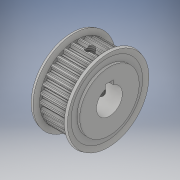
# Autodesk Inventor part: HTPA30S3M100-A-N10_b
Saved by Autodesk Inventor 2019 (Build 230136000, 136)
## iProperties
Created: 2022-11-15
Part Number: HTPA30S3M100-A-N10_b
Material: Generic
Catalog Web Link: www.cadenas.de
Description: HTPA__S3M060, HTPA__S3M100, HTPA__S3M150, HTPB__S3M060, HTPB__S3M100, HTPB__S3M150, HTPK__S3M060, HTPK__S3M100, HTPK__S3M150, HTPN__S3M060, HTPN__S3M100, HTPN__S3M150, HTPT__S3M060, HTPT__S3M100, HTPT__S3M150, HTPM__S3M060, HTPM__S3M100, HTPM__S3M150, HTPP__S3M060, HTPP__S3M100, HTPP__S3M150, HTPS__S3M060, HTPS__S3M100, KHTPA__S3M060, KHTPA__S3M100, KHTPA__S3M150, KHTPK__S3M060, KHTPK__S3M100, KHTPK__S3M150_body-High Torque Timing Pulleys S3M Type
Vendor: MISUMI
Document SubType Name: Modeling
Designer: psAdmin
Manufacturer: MISUMI
Mass: 7.23105 g
Surface Area: 42.2616 cm^2
Volume: 7.23105 cm^3
Density: 1 g/cm^3
Appearance: PSOLRGB-175-175-175
Category: PARTsolutions
Company: MISUMI
Title: HTPA30S3M100-A-N10
Author: Cadenas PARTsolutions
Comments: High Torque Timing Pulleys S3M Type
PSOL_IDENT_0: {$CADENAS_DATA/23d-libs/misumi/metric/51_timing_pulleys/htpk_s3m/htpa_s3m.prj},837 {VTYP=3D},{NB=HTP
PSOL_IDENT_1: A30S3M100-A-N10_b},{LINA=HTPA30S3M100-A-N10},{NN=HTPA__S3M060, HTPA__S3M100, HTPA__S3M150, HTPB__S3M
PSOL_IDENT_2: 060, HTPB__S3M100, HTPB__S3M150, HTPK__S3M060, HTPK__S3M100, HTPK__S3M150, HTPN__S3M060, HTPN__S3M10
PSOL_IDENT_3: 0, HTPN__S3M150, HTPT__S3M060, HTPT__S3M100, HTPT__S3M150, HTPM__S3M060, HTPM__S3M100, HTPM__S3M150,
PSOL_IDENT_4: HTPP__S3M060, HTPP__S3M100, HTPP__S3M150, HTPS__S3M060, HTPS__S3M100, KHTPA__S3M060, KHTPA__S3M100,
PSOL_IDENT_5: KHTPA__S3M150, KHTPK__S3M060, KHTPK__S3M100, KHTPK__S3M150_body},{DATE=28.10.2022 00:10:57},{GEOMDA
PSOL_IDENT_6: TE=11.11.2021 09:52:43},{VERSION=},{LINEID=160},{WBVAR=MATP,ST,TNW,PS,SBS,DD,Z,J,Q,R,S,T,ALT1,ALT2,M
PSOL_IDENT_7: ,QSC,QFC,QTC,ALT3,K,KSC,KFC,KTC,ALT4,ZM,ZSC,ZFC,ZTC,ALT5,ALT6,ALT7,FC,ALT8,SRG,ALT9,BTC,TL,ALT10,TPC
PSOL_IDENT_8: ,ALT11,BC,ALT12,SLH,ALT13,BN},{WBNUMERIC=DD,Z,J,Q,R,S,T,QSC,QFC,QTC,K,KSC,KFC,KTC,ZSC,ZFC,ZTC,FC,SRG
PSOL_IDENT_9: ,BTC,TL,BC,SLH,BN}  {NB=HTPA30S3M100-A-N10_b},{LINA=HTPA30S3M100-A-N10},{KT=DUMMY},{PN=HTPA30S3M100-
PSOL_IDENT_10: A-N10},{TYPE=HTPA},{MATP=A2017},{MATPALG='A2017','Aluminum Alloy 2000 series','S45C','1045 Carbon St
PSOL_IDENT_11: eel Equivalent','SUS304','304 Stainless Steel','A6000','6000 Series Aluminum Alloy'},{ST=CA},{STALG=
PSOL_IDENT_12: 'CA','Clear Anodize','BA','Black Anodize','HAT','Hard Clear Anodize','ENP','Electroless Nickel Plat
PSOL_IDENT_13: ing' },{NT=30},{TNW=S3M100},{TNWALG= 'S3M060','S3M100','S3M150'    },{BW=10},{PS=A},{PSALG='A','B'},
PSOL_IDENT_14: {SBS=N},{SBSALG= 'H','Round Hole','P','Round Hole + Tap','N','New JIS Keywayed Bore + Tap (Standard)'
PSOL_IDENT_15: ,'NK','New JIS Keywayed Bore + Tap (width 4.0mm, height 1.8mm)','C','Old JIS Keywayed Bore + Tap','V'
PSOL_IDENT_16: ,'Stepped Hole', 'Y','Both Ends Stepped Hole','WB', 'Double Stepped Hole' },{SHSA= 'H','Round Hole','
PSOL_IDENT_17: P','Round Hole + Tap','N','New JIS Keywayed Bore + Tap (Standard)','NK','New JIS Keywayed Bore + Tap
PSOL_IDENT_18: (width 4.0mm, height 1.8mm)','C','Old JIS Keywayed Bore + Tap','V','Stepped Hole', 'Y','Both Ends S
PSOL_IDENT_19: tepped Hole','WB', 'Double Stepped Hole' },{SHSB= 'H','Round Hole','P','Round Hole + Tap','N','New J
PSOL_IDENT_20: IS Keywayed Bore + Tap (Standard)','NK','New JIS Keywayed Bore + Tap (width 4.0mm, height 1.8mm)','C'
PSOL_IDENT_21: ,'Old JIS Keywayed Bore + Tap','V','Stepped Hole', 'F','Stepped Hole (Counterbore holes on the boss
PSOL_IDENT_22: side)'},{SHSK= '','' },{SBSPN=-N10},{DD=10.00},{DDALG=[8:8/1],[10:14/1]},{DDHA=[6:6/1],6.35,[7:12/1]
PSOL_IDENT_23: ,12.7,[13:19/1]},{DDHBK=0},{DDPA=[6:6/1],6.35,[7:12/1],12.7,[13:19/1]},{DDPBK=0},{DDNA=[8:8/1],[10:1
PSOL_IDENT_24: 4/1]},{DDNBK=0},{DDNK=10},{DDCA=[10:10/1],[12:12/1]},{DDCBK=0},{DDVA=[6:6/1],6.35,[7:12/1],12.7,[13:
PSOL_IDENT_25: 17/1]},{DDVF=[6:6/1],6.35,[7:12/1],12.7,[13:14/1]},{DDY=[6:17/1]},{DDWB=[6:15/1]},{Z=0},{ZALG=[0]},{
PSOL_IDENT_26: ZQRMIN=12},{ZAMAX=19},{ZBMAX=16},{DDZ=10},{J=0.0},{JALG=[0]},{JMAX=13},{JMIN=2},{JPN=},{QRMAX=19},{Q
PSOL_IDENT_27: RMIN=12},{WBRMAX=-2.00},{WBQMIN=14},{Q=0},{QALG=[0]},{QPN=},{R=0},{RALG=[0]},{S=0.0},{SALG=[0]},{SPN=
PSOL_IDENT_28: },{SMAX=9},{T=0.0},{TALG=[0]},{TPN=},{TMAX=12},{A=11},{W=15},{L=0},{PD=28.65},{OD=27.89},{D=0},{DALG=
PSOL_IDENT_29: 20},{DE=23},{F=32},{E=23},{BBK=3.000},{TTK=1.4},{TT=1},{ANG=120},{WL=15},{ALT1=},{ALT1ALG= '','w/o K
PSOL_IDENT_30: C90 (Set Screw Angle)','KC90','with KC90 (Set Screw Angle)' },{ALT1PN=},{ALT2=},{ALT2ALG= '','Not ap
PSOL_IDENT_31: plicable' },{M=N/A},{MALG= 'N/A' },{MFTALG= 'N/A' },{MSALG= 'N/A' },{M3D=0.000},{KDML=0},{ML=0},{MUL=
PSOL_IDENT_32: 0},{PITCH=0},{QSC=0.0},{QSCALG=0},{QFC=0.0},{QFCALG=0},{QTC=0.0},{QTCALG=0},{QPCDMIN=0},{QPCDMINALG=
PSOL_IDENT_33: 0},{QPCDMAX=19},{ALT2PN=},{ALT3=},{ALT3ALG= '','Not applicable' },{K=0.0},{KALG=0},{KMIN=4},{KFTMAX=
PSOL_IDENT_34: 0.0},{KSMAX=0.0},{KSC=0.0},{KSCALG=0},{KFC=0.0},{KFCALG=0},{KTC=0.0},{KTCALG=0},{KPCDMIN=14},{KPCDMI
PSOL_IDENT_35: NALG=14},{KPCDMAX=19},{KSCMIN=14.0},{KSCMINALG=14},{ALT3PN=},{ALT4=},{ALT4ALG= '','Not applicable' }
PSOL_IDENT_36: ,{ALT4MIN=20.5},{ALT4MAX=12.5},{ZM=N/A},{ZMALG= 'N/A' },{ZMSALG= 'N/A' },{ZMFTALG= 'N/A' },{ZMDD1=0.
PSOL_IDENT_37: 0},{ZMDD2=0.0},{ZMHH=0.0},{ZSC=0.0},{ZSCALG=[0]},{ZFC=0.0},{ZFCALG=[0]},{ZTC=0.0},{ZTCALG=[0]},{ZPCD
PSOL_IDENT_38: MIN=0},{ZPCDMINALG=0},{ZPCDMAX=19},{ALT4PN=},{ALT5=},{ALT5ALG= '','Flange Attached','NFC','with NFC
PSOL_IDENT_39: (Flange not Attached)' },{ALT5PN=},{ALT6=},{ALT6ALG= '','w/o Flange Attached on One Side Only','RFC'
PSOL_IDENT_40: ,'with RFC (Flange Attached on The Boss Side Only)','LFC','with LFC (Flange Attached on The Opposite
PSOL_IDENT_41: Side Only)' },{ALT6PN=},{ALT7=},{ALT7ALG= '','w/o FC (Flange Cut)','FC','with FC (Flange Cut)' },{F
PSOL_IDENT_42: C=0.0},{FCALG=0},{FCMIN=29.0},{FCMAX=30.0},{ALT7PN=},{ALT8=},{ALT8ALG= '','Not applicable' },{ALT8AL
PSOL_IDENT_43: GALG=19},{ALT8DD2=0},{ALT8MM=0},{ALT8NN=0},{QC=0},{KC=0},{ZC=0},{SRG=0.0},{SRGALG=[0]},{SRGMAX1=0},{
PSOL_IDENT_44: SRGMAX=0},{DD2=0.0},{MM=0.00},{NN=0.00},{ALT8PN=},{ALT9ALG= '','Not applicable' },{ALT9=},{BTC9=11},
PSOL_IDENT_45: {TL9=1},{BTC=0},{BTCALG=[0]},{TL=0.0},{TLALG=0},{TLMIN=1.0},{TLMAX=-15.5},{BTCL=0},{BTCD=0},{BTCDALG=
PSOL_IDENT_46: 20.000},{ALT9PN=},{WLBCTL=15},{ALT10=},{ALT10ALG= '','w/o TPC (Tapped Hole Dimension)','TPC','with T
PSOL_IDENT_47: PC (Tapped Hole Dimension)' },{TPC=N/A},{TPCALG= 'N/A' },{TPCM=4},{ALT10PN=},{ALT11=},{ALT11ALG= '','
PSOL_IDENT_48: Not applicable' },{BC=0.0},{BCALG=0},{BCMIN=7},{BCMAX=-15.5},{BCPLANE=7.5},{M1WBC=7.5},{ALT11PN=},{A
PSOL_IDENT_49: LT12=},{ALT12ALG= '','w/o SLH (Set Screw Length)','SLH','with SLH (Set Screw Length)' },{SLH=0},{SLH
PSOL_IDENT_50: ALG=[0]},{ALT12PN=},{AC=M4x3},{M1=4},{M1L=3},{TAP=0.000},{KYY=5},{KTT=8.945},{PLANE=15},{CD=0},{ALT1
PSOL_IDENT_51: 3=},{ALT13ALG= '', 'Not applicable' },{BN=0.0},{BNALG=0},{BNMIN=-14.5},{BNMAX=-5.0},{ALT13PN=}
NB: HTPA30S3M100-A-N10_b
NN: 0
NT: 30
NBSYN: $PN._b
LINA: HTPA30S3M100-A-N10
CATALOG: Misumi
PN: HTPA30S3M100-A-N10
MATP: Aluminum Alloy 2000 series
ST: Clear Anodize
TNW: S3M100
BW: 10
PS: A
SBS: New JIS Keywayed Bore + Tap (Standard)
DD: 10
Z: 0
J: 0
Q: 0
R: 0
S: 0
T: 0
A: 11
W: 15
L: 0
PD: 28.65
OD: 27.89
D: 0
F: 32
E: 23
TT: 1
ALT1: w/o KC90 (Set Screw Angle)
ALT2: Not applicable
M: N/A
QSC: 0
QFC: 0
QTC: 0
ALT3: Not applicable
K: 0
KSC: 0
KFC: 0
KTC: 0
ALT4: Not applicable
ZM: N/A
ZMDD1: 0
ZMDD2: 0
ZMHH: 0
ZSC: 0
ZFC: 0
ZTC: 0
ALT5: Flange Attached
ALT6: w/o Flange Attached on One Side Only
ALT7: w/o FC (Flange Cut)
FC: 0
ALT8: Not applicable
SRG: 0
DD2: 0
MM: 0
ALT9: Not applicable
BTC: 0
TL: 0
BTCL: 0
BTCD: 0
ALT10: w/o TPC (Tapped Hole Dimension)
TPC: N/A
ALT11: Not applicable
BC: 0
ALT12: w/o SLH (Set Screw Length)
SLH: 0
AC: M4x3
ALT13: Not applicable
BN: 0
SUPPLIER: MISUMI
ARTICLENO: HTPA30S3M100-A-N10_b
BOMINFO: HTPA30S3M100-A-N10
CREATOR: CADENAS GmbH
Autodesk Inventor part; units mm, degrees
sketch "_____1" plane through (0, 0, 0) normal (0, 0, 1) x (1, 0, 0)
  line L0 (15, 0) -> (0, 0)
  line L1 (0, 0) -> (0, 11.5)
  line L2 (0, 11.5) -> (1, 11.5)
  line L3 (1, 11.5) -> (1, 13.813348)
  line L4 (1, 13.813348) -> (0.483439, 15.741181)
  line L5 (0.483439, 15.741181) -> (1.449364, 16)
  line L6 (1.449364, 16) -> (2, 13.945)
  line L7 (2, 13.945) -> (13, 13.945)
  line L8 (13, 13.945) -> (13.550636, 16)
  line L9 (13.550636, 16) -> (14.516561, 15.741181)
  line L10 (14.516561, 15.741181) -> (14, 13.813348)
  line L11 (14, 13.813348) -> (14, 11.5)
  line L12 (14, 11.5) -> (15, 11.5)
  line L13 (15, 11.5) -> (15, 0)
  line L14 (15, 0) -> (0, 0)
  constraints: 30 end point
revolve "Revolution1" add sketch "_____1" angle 360 about axis through (15, 0, 0) along (1, 0, 0)
sketch "Sketch2" plane through (15, 0, 0) normal (1, 0, 0) x (0, 0, -1)
  point P0 (0, 0)
hole "Hole1" at (15, 0, 0) direction (-1, 0, 0) diameter 10 depth 15
sketch "_____6" plane through (2, 0, 0) normal (1, 0, 0) x (0, 0, -1)
  circle A0 centre (0, 0) radius 18.945
  arc A1 (-13.942597, 0.258894) -> (-13.942597, -0.258894) centre (0, 0) ccw
  arc A2 (-13.942597, -0.258894) -> (-13.718388, -0.52809) centre (-13.662645, -0.253695) ccw
  arc A3 (-12.845232, -0.94797) -> (-13.718388, -0.52809) centre (-14.111574, -2.463557) ccw
  arc A4 (-12.791913, -1.050797) -> (-12.845232, -0.94797) centre (-12.94141, -1.063078) ccw
  arc A5 (-12.791913, -1.050797) -> (-12.730852, -1.631754) centre (0, 0) ccw
  arc A6 (-12.761627, -1.74342) -> (-12.730852, -1.631754) centre (-12.879635, -1.650824) ccw
  arc A7 (-13.528404, -2.335663) -> (-12.761627, -1.74342) centre (-14.315404, -0.524239) ccw
  arc A8 (-13.528404, -2.335663) -> (-13.691744, -2.645593) centre (-13.416829, -2.592472) ccw
  arc A9 (-13.691744, -2.645593) -> (-13.58409, -3.152065) centre (0, 0) ccw
  arc A10 (-13.58409, -3.152065) -> (-13.308812, -3.368764) centre (-13.311337, -3.088775) ccw
  arc A11 (-12.367439, -3.597928) -> (-13.308812, -3.368764) centre (-13.291, -5.343683) ccw
  arc A12 (-12.293906, -3.687423) -> (-12.367439, -3.597928) centre (-12.437583, -3.730517) ccw
  arc A13 (-12.293906, -3.687423) -> (-12.113392, -4.242989) centre (0, 0) ccw
  arc A14 (-12.120277, -4.358613) -> (-12.113392, -4.242989) centre (-12.254959, -4.292576) ccw
  arc A15 (-12.747165, -5.097336) -> (-12.120277, -4.358613) centre (-13.893583, -3.489123) ccw
  arc A16 (-12.747165, -5.097336) -> (-12.842497, -5.434454) centre (-12.584634, -5.325336) ccw
  arc A17 (-12.842497, -5.434454) -> (-12.631894, -5.907476) centre (0, 0) ccw
  arc A18 (-12.631894, -5.907476) -> (-12.317577, -6.062206) centre (-12.37826, -5.78886) ccw
  arc A19 (-11.349129, -6.09064) -> (-12.317577, -6.062206) centre (-11.889545, -7.990265) ccw
  arc A20 (-11.258597, -6.162891) -> (-11.349129, -6.09064) centre (-11.390174, -6.234915) ccw
  arc A21 (-11.258597, -6.162891) -> (-10.966518, -6.668785) centre (0, 0) ccw
  arc A22 (-10.949214, -6.783314) -> (-10.966518, -6.668785) centre (-11.094682, -6.746722) ccw
  arc A23 (-11.408813, -7.636232) -> (-10.949214, -6.783314) centre (-12.864545, -6.301516) ccw
  arc A24 (-11.408813, -7.636232) -> (-11.431971, -7.985803) centre (-11.20243, -7.825457) ccw
  arc A25 (-11.431971, -7.985803) -> (-11.127624, -8.404702) centre (0, 0) ccw
  arc A26 (-11.127624, -8.404702) -> (-10.788005, -8.4907) centre (-10.904194, -8.235945) ccw
  arc A27 (-9.834808, -8.317162) -> (-10.788005, -8.4907) centre (-9.968461, -10.287634) ccw
  arc A28 (-9.731232, -8.369011) -> (-9.834808, -8.317162) centre (-9.844959, -8.466818) ccw
  arc A29 (-9.731232, -8.369011) -> (-9.340355, -8.803124) centre (0, 0) ccw
  arc A30 (-9.299617, -8.911552) -> (-9.340355, -8.803124) centre (-9.449514, -8.906004) ccw
  arc A31 (-9.571841, -9.841387) -> (-9.299617, -8.911552) centre (-11.273265, -8.838502) ccw
  arc A32 (-9.571841, -9.841387) -> (-9.521814, -10.188135) centre (-9.330626, -9.983569) ccw
  arc A33 (-9.521814, -10.188135) -> (-9.137023, -10.534602) centre (0, 0) ccw
  arc A34 (-9.137023, -10.534602) -> (-8.786945, -10.54811) centre (-8.953562, -10.323079) ccw
  arc A35 (-7.890659, -10.180183) -> (-8.786945, -10.54811) centre (-7.611706, -12.135384) ccw
  arc A36 (-7.778566, -10.209365) -> (-7.890659, -10.180183) centre (-7.869473, -10.32868) ccw
  arc A37 (-7.778566, -10.209365) -> (-7.305974, -10.552723) centre (0, 0) ccw
  arc A38 (-7.243582, -10.650312) -> (-7.305974, -10.552723) centre (-7.391357, -10.676051) ccw
  arc A39 (-7.316534, -11.616427) -> (-7.243582, -10.650312) centre (-9.18929, -10.989203) ccw
  arc A40 (-7.316534, -11.616427) -> (-7.195507, -11.945196) centre (-7.051029, -11.70535) ccw
  arc A41 (-7.195507, -11.945196) -> (-6.74709, -12.20409) centre (0, 0) ccw
  arc A42 (-6.74709, -12.20409) -> (-6.401854, -12.144517) centre (-6.611616, -11.959045) ccw
  arc A43 (-5.60165, -11.598282) -> (-6.401854, -12.144517) centre (-4.922284, -13.45276) ccw
  arc A44 (-5.48594, -11.603521) -> (-5.60165, -11.598282) centre (-5.550053, -11.739129) ccw
  arc A45 (-5.48594, -11.603521) -> (-4.952286, -11.841118) centre (0, 0) ccw
  arc A46 (-4.870968, -11.923603) -> (-4.952286, -11.841118) centre (-5.010163, -11.979503) ccw
  arc A47 (-4.741459, -12.883773) -> (-4.870968, -11.923603) centre (-6.703698, -12.659623) ccw
  arc A48 (-4.741459, -12.883773) -> (-4.554722, -13.180195) centre (-4.463268, -12.915551) ccw
  arc A49 (-4.554722, -13.180195) -> (-4.062277, -13.3402) centre (0, 0) ccw
  arc A50 (-4.062277, -13.3402) -> (-3.736971, -13.210151) centre (-3.980711, -13.072344) ccw
  arc A51 (-3.067822, -12.50948) -> (-3.736971, -13.210151) centre (-2.017734, -14.182185) ccw
  arc A52 (-2.953551, -12.490547) -> (-3.067822, -12.50948) centre (-2.988069, -12.636521) ccw
  arc A53 (-2.953551, -12.490547) -> (-2.38216, -12.612) centre (0, 0) ccw
  arc A54 (-2.285469, -12.675775) -> (-2.38216, -12.612) centre (-2.41, -12.759394) ccw
  arc A55 (-1.959159, -13.588036) -> (-2.285469, -12.675775) centre (-3.925122, -13.776757) ccw
  arc A56 (-1.959159, -13.588036) -> (-1.714874, -13.839156) centre (-1.680441, -13.561281) ccw
  arc A57 (-1.714874, -13.839156) -> (-1.199923, -13.893279) centre (0, 0) ccw
  arc A58 (-1.199923, -13.893279) -> (-0.908764, -13.698437) centre (-1.17583, -13.614318) ccw
  arc A59 (-0.399916, -12.873954) -> (-0.908764, -13.698437) centre (0.975, -14.291781) ccw
  arc A60 (-0.292078, -12.831676) -> (-0.399916, -12.873954) centre (-0.295492, -12.981637) ccw
  arc A61 (-0.292078, -12.831676) -> (0.292078, -12.831676) centre (0, 0) ccw
  arc A62 (0.399916, -12.873954) -> (0.292078, -12.831676) centre (0.295492, -12.981637) ccw
  arc A63 (0.908764, -13.698437) -> (0.399916, -12.873954) centre (-0.975, -14.291781) ccw
  arc A64 (0.908764, -13.698437) -> (1.199923, -13.893279) centre (1.17583, -13.614318) ccw
  arc A65 (1.199923, -13.893279) -> (1.714873, -13.839156) centre (0, 0) ccw
  arc A66 (1.714873, -13.839156) -> (1.95916, -13.588036) centre (1.680441, -13.561281) ccw
  arc A67 (2.285469, -12.675775) -> (1.95916, -13.588036) centre (3.925122, -13.776757) ccw
  arc A68 (2.38216, -12.612) -> (2.285469, -12.675775) centre (2.41, -12.759394) ccw
  arc A69 (2.38216, -12.612) -> (2.953551, -12.490547) centre (0, 0) ccw
  arc A70 (3.067822, -12.50948) -> (2.953551, -12.490547) centre (2.988069, -12.636521) ccw
  arc A71 (3.736971, -13.210151) -> (3.067822, -12.50948) centre (2.017734, -14.182185) ccw
  arc A72 (3.736971, -13.210151) -> (4.062277, -13.3402) centre (3.980711, -13.072344) ccw
  arc A73 (4.062277, -13.3402) -> (4.554722, -13.180195) centre (0, 0) ccw
  arc A74 (4.554722, -13.180195) -> (4.741459, -12.883773) centre (4.463268, -12.915551) ccw
  arc A75 (4.870968, -11.923603) -> (4.741459, -12.883773) centre (6.703698, -12.659623) ccw
  arc A76 (4.952286, -11.841118) -> (4.870968, -11.923603) centre (5.010163, -11.979503) ccw
  arc A77 (4.952286, -11.841118) -> (5.48594, -11.603521) centre (0, 0) ccw
  arc A78 (5.60165, -11.598282) -> (5.48594, -11.603521) centre (5.550053, -11.739129) ccw
  arc A79 (6.401854, -12.144518) -> (5.60165, -11.598282) centre (4.922284, -13.45276) ccw
  arc A80 (6.401854, -12.144518) -> (6.74709, -12.20409) centre (6.611616, -11.959045) ccw
  arc A81 (6.74709, -12.20409) -> (7.195507, -11.945196) centre (0, 0) ccw
  arc A82 (7.195507, -11.945196) -> (7.316534, -11.616427) centre (7.051029, -11.70535) ccw
  arc A83 (7.243582, -10.650312) -> (7.316534, -11.616427) centre (9.18929, -10.989203) ccw
  arc A84 (7.305974, -10.552723) -> (7.243582, -10.650312) centre (7.391357, -10.676051) ccw
  arc A85 (7.305974, -10.552723) -> (7.778566, -10.209365) centre (0, 0) ccw
  arc A86 (7.890659, -10.180183) -> (7.778566, -10.209365) centre (7.869473, -10.32868) ccw
  arc A87 (8.786945, -10.54811) -> (7.890659, -10.180183) centre (7.611706, -12.135384) ccw
  arc A88 (8.786945, -10.54811) -> (9.137023, -10.534602) centre (8.953562, -10.323079) ccw
  arc A89 (9.137023, -10.534602) -> (9.521813, -10.188135) centre (0, 0) ccw
  arc A90 (9.521813, -10.188135) -> (9.571841, -9.841387) centre (9.330626, -9.983569) ccw
  arc A91 (9.299617, -8.911552) -> (9.571841, -9.841387) centre (11.273265, -8.838502) ccw
  arc A92 (9.340355, -8.803124) -> (9.299617, -8.911552) centre (9.449514, -8.906004) ccw
  arc A93 (9.340355, -8.803124) -> (9.731232, -8.369011) centre (0, 0) ccw
  arc A94 (9.834808, -8.317162) -> (9.731232, -8.369011) centre (9.844959, -8.466818) ccw
  arc A95 (10.788005, -8.4907) -> (9.834808, -8.317162) centre (9.968461, -10.287634) ccw
  arc A96 (10.788005, -8.4907) -> (11.127624, -8.404702) centre (10.904194, -8.235945) ccw
  arc A97 (11.127624, -8.404702) -> (11.431971, -7.985803) centre (0, 0) ccw
  arc A98 (11.431971, -7.985803) -> (11.408813, -7.636232) centre (11.20243, -7.825457) ccw
  arc A99 (10.949214, -6.783314) -> (11.408813, -7.636232) centre (12.864545, -6.301516) ccw
  arc A100 (10.966518, -6.668785) -> (10.949214, -6.783314) centre (11.094682, -6.746722) ccw
  arc A101 (10.966518, -6.668785) -> (11.258597, -6.162891) centre (0, 0) ccw
  arc A102 (11.349129, -6.09064) -> (11.258597, -6.162891) centre (11.390174, -6.234915) ccw
  arc A103 (12.317577, -6.062206) -> (11.349129, -6.09064) centre (11.889545, -7.990265) ccw
  arc A104 (12.317577, -6.062206) -> (12.631894, -5.907476) centre (12.37826, -5.78886) ccw
  arc A105 (12.631894, -5.907476) -> (12.842497, -5.434454) centre (0, 0) ccw
  arc A106 (12.842497, -5.434454) -> (12.747164, -5.097336) centre (12.584634, -5.325336) ccw
  arc A107 (12.120277, -4.358613) -> (12.747164, -5.097336) centre (13.893583, -3.489123) ccw
  arc A108 (12.113392, -4.242989) -> (12.120277, -4.358613) centre (12.254959, -4.292576) ccw
  arc A109 (12.113392, -4.242989) -> (12.293906, -3.687423) centre (0, 0) ccw
  arc A110 (12.367439, -3.597928) -> (12.293906, -3.687423) centre (12.437583, -3.730517) ccw
  arc A111 (13.308812, -3.368764) -> (12.367439, -3.597928) centre (13.291, -5.343683) ccw
  arc A112 (13.308812, -3.368764) -> (13.58409, -3.152065) centre (13.311337, -3.088775) ccw
  arc A113 (13.58409, -3.152065) -> (13.691744, -2.645593) centre (0, 0) ccw
  arc A114 (13.691744, -2.645593) -> (13.528404, -2.335663) centre (13.416829, -2.592472) ccw
  arc A115 (12.761627, -1.74342) -> (13.528404, -2.335663) centre (14.315404, -0.524239) ccw
  arc A116 (12.730852, -1.631754) -> (12.761627, -1.74342) centre (12.879635, -1.650824) ccw
  arc A117 (12.730852, -1.631754) -> (12.791913, -1.050797) centre (0, 0) ccw
  arc A118 (12.845232, -0.94797) -> (12.791913, -1.050797) centre (12.94141, -1.063078) ccw
  arc A119 (13.718388, -0.52809) -> (12.845232, -0.94797) centre (14.111574, -2.463557) ccw
  arc A120 (13.718388, -0.52809) -> (13.942597, -0.258894) centre (13.662645, -0.253695) ccw
  arc A121 (13.942597, -0.258894) -> (13.942597, 0.258894) centre (0, 0) ccw
  arc A122 (13.942597, 0.258894) -> (13.718388, 0.52809) centre (13.662645, 0.253695) ccw
  arc A123 (12.845232, 0.94797) -> (13.718388, 0.52809) centre (14.111574, 2.463557) ccw
  arc A124 (12.791913, 1.050797) -> (12.845232, 0.94797) centre (12.94141, 1.063078) ccw
  arc A125 (12.791913, 1.050797) -> (12.730852, 1.631754) centre (0, 0) ccw
  arc A126 (12.761627, 1.74342) -> (12.730852, 1.631754) centre (12.879635, 1.650824) ccw
  arc A127 (13.528404, 2.335663) -> (12.761627, 1.74342) centre (14.315404, 0.524239) ccw
  arc A128 (13.528404, 2.335663) -> (13.691744, 2.645593) centre (13.416829, 2.592472) ccw
  arc A129 (13.691744, 2.645593) -> (13.58409, 3.152065) centre (0, 0) ccw
  arc A130 (13.58409, 3.152065) -> (13.308812, 3.368764) centre (13.311337, 3.088775) ccw
  arc A131 (12.367439, 3.597928) -> (13.308812, 3.368764) centre (13.291, 5.343683) ccw
  arc A132 (12.293906, 3.687423) -> (12.367439, 3.597928) centre (12.437583, 3.730517) ccw
  arc A133 (12.293906, 3.687423) -> (12.113392, 4.242989) centre (0, 0) ccw
  arc A134 (12.120277, 4.358613) -> (12.113392, 4.242989) centre (12.254959, 4.292576) ccw
  arc A135 (12.747165, 5.097336) -> (12.120277, 4.358613) centre (13.893583, 3.489123) ccw
  arc A136 (12.747165, 5.097336) -> (12.842497, 5.434454) centre (12.584634, 5.325336) ccw
  arc A137 (12.842497, 5.434454) -> (12.631894, 5.907476) centre (0, 0) ccw
  arc A138 (12.631894, 5.907476) -> (12.317577, 6.062206) centre (12.37826, 5.78886) ccw
  arc A139 (11.349129, 6.09064) -> (12.317577, 6.062206) centre (11.889545, 7.990265) ccw
  arc A140 (11.258597, 6.162891) -> (11.349129, 6.09064) centre (11.390174, 6.234915) ccw
  arc A141 (11.258597, 6.162891) -> (10.966518, 6.668785) centre (0, 0) ccw
  arc A142 (10.949214, 6.783314) -> (10.966518, 6.668785) centre (11.094682, 6.746722) ccw
  arc A143 (11.408812, 7.636232) -> (10.949214, 6.783314) centre (12.864545, 6.301516) ccw
  arc A144 (11.408812, 7.636232) -> (11.431971, 7.985803) centre (11.20243, 7.825457) ccw
  arc A145 (11.431971, 7.985803) -> (11.127624, 8.404702) centre (0, 0) ccw
  arc A146 (11.127624, 8.404702) -> (10.788005, 8.4907) centre (10.904194, 8.235945) ccw
  arc A147 (9.834808, 8.317162) -> (10.788005, 8.4907) centre (9.968461, 10.287634) ccw
  arc A148 (9.731232, 8.369011) -> (9.834808, 8.317162) centre (9.844959, 8.466818) ccw
  arc A149 (9.731232, 8.369011) -> (9.340355, 8.803124) centre (0, 0) ccw
  arc A150 (9.299617, 8.911552) -> (9.340355, 8.803124) centre (9.449514, 8.906004) ccw
  arc A151 (9.571841, 9.841387) -> (9.299617, 8.911552) centre (11.273265, 8.838502) ccw
  arc A152 (9.571841, 9.841387) -> (9.521814, 10.188135) centre (9.330626, 9.983569) ccw
  arc A153 (9.521814, 10.188135) -> (9.137023, 10.534602) centre (0, 0) ccw
  arc A154 (9.137023, 10.534602) -> (8.786945, 10.54811) centre (8.953562, 10.323079) ccw
  arc A155 (7.890659, 10.180183) -> (8.786945, 10.54811) centre (7.611706, 12.135384) ccw
  arc A156 (7.778566, 10.209365) -> (7.890659, 10.180183) centre (7.869473, 10.32868) ccw
  arc A157 (7.778566, 10.209365) -> (7.305974, 10.552723) centre (0, 0) ccw
  arc A158 (7.243582, 10.650312) -> (7.305974, 10.552723) centre (7.391357, 10.676051) ccw
  arc A159 (7.316534, 11.616427) -> (7.243582, 10.650312) centre (9.18929, 10.989203) ccw
  arc A160 (7.316534, 11.616427) -> (7.195507, 11.945196) centre (7.051029, 11.70535) ccw
  arc A161 (7.195507, 11.945196) -> (6.74709, 12.20409) centre (0, 0) ccw
  arc A162 (6.74709, 12.20409) -> (6.401854, 12.144517) centre (6.611616, 11.959045) ccw
  arc A163 (5.60165, 11.598282) -> (6.401854, 12.144517) centre (4.922284, 13.45276) ccw
  arc A164 (5.48594, 11.603521) -> (5.60165, 11.598282) centre (5.550053, 11.739129) ccw
  arc A165 (5.48594, 11.603521) -> (4.952286, 11.841118) centre (0, 0) ccw
  arc A166 (4.870968, 11.923603) -> (4.952286, 11.841118) centre (5.010163, 11.979503) ccw
  arc A167 (4.741459, 12.883773) -> (4.870968, 11.923603) centre (6.703698, 12.659623) ccw
  arc A168 (4.741459, 12.883773) -> (4.554722, 13.180195) centre (4.463268, 12.915551) ccw
  arc A169 (4.554722, 13.180195) -> (4.062277, 13.3402) centre (0, 0) ccw
  arc A170 (4.062277, 13.3402) -> (3.736971, 13.210151) centre (3.980711, 13.072344) ccw
  arc A171 (3.067822, 12.50948) -> (3.736971, 13.210151) centre (2.017734, 14.182185) ccw
  arc A172 (2.953551, 12.490547) -> (3.067822, 12.50948) centre (2.988069, 12.636521) ccw
  arc A173 (2.953551, 12.490547) -> (2.38216, 12.612) centre (0, 0) ccw
  arc A174 (2.285469, 12.675775) -> (2.38216, 12.612) centre (2.41, 12.759394) ccw
  arc A175 (1.95916, 13.588036) -> (2.285469, 12.675775) centre (3.925122, 13.776757) ccw
  arc A176 (1.95916, 13.588036) -> (1.714873, 13.839156) centre (1.680441, 13.561281) ccw
  arc A177 (1.714873, 13.839156) -> (1.199923, 13.893279) centre (0, 0) ccw
  arc A178 (1.199923, 13.893279) -> (0.908764, 13.698437) centre (1.17583, 13.614318) ccw
  arc A179 (0.399916, 12.873954) -> (0.908764, 13.698437) centre (-0.975, 14.291781) ccw
  arc A180 (0.292078, 12.831676) -> (0.399916, 12.873954) centre (0.295492, 12.981637) ccw
  arc A181 (0.292078, 12.831676) -> (-0.292078, 12.831676) centre (0, 0) ccw
  arc A182 (-0.399916, 12.873954) -> (-0.292078, 12.831676) centre (-0.295492, 12.981637) ccw
  arc A183 (-0.908764, 13.698437) -> (-0.399916, 12.873954) centre (0.975, 14.291781) ccw
  arc A184 (-0.908764, 13.698437) -> (-1.199923, 13.893279) centre (-1.17583, 13.614318) ccw
  arc A185 (-1.199923, 13.893279) -> (-1.714873, 13.839156) centre (0, 0) ccw
  arc A186 (-1.714873, 13.839156) -> (-1.95916, 13.588036) centre (-1.680441, 13.561281) ccw
  arc A187 (-2.285469, 12.675775) -> (-1.95916, 13.588036) centre (-3.925122, 13.776757) ccw
  arc A188 (-2.38216, 12.612) -> (-2.285469, 12.675775) centre (-2.41, 12.759394) ccw
  arc A189 (-2.38216, 12.612) -> (-2.953551, 12.490547) centre (0, 0) ccw
  arc A190 (-3.067822, 12.50948) -> (-2.953551, 12.490547) centre (-2.988069, 12.636521) ccw
  arc A191 (-3.736971, 13.210151) -> (-3.067822, 12.50948) centre (-2.017734, 14.182185) ccw
  arc A192 (-3.736971, 13.210151) -> (-4.062277, 13.3402) centre (-3.980711, 13.072344) ccw
  arc A193 (-4.062277, 13.3402) -> (-4.554722, 13.180195) centre (0, 0) ccw
  arc A194 (-4.554722, 13.180195) -> (-4.741459, 12.883773) centre (-4.463268, 12.915551) ccw
  arc A195 (-4.870968, 11.923603) -> (-4.741459, 12.883773) centre (-6.703698, 12.659623) ccw
  arc A196 (-4.952286, 11.841118) -> (-4.870968, 11.923603) centre (-5.010163, 11.979503) ccw
  arc A197 (-4.952286, 11.841118) -> (-5.48594, 11.603521) centre (0, 0) ccw
  arc A198 (-5.60165, 11.598282) -> (-5.48594, 11.603521) centre (-5.550053, 11.739129) ccw
  arc A199 (-6.401854, 12.144517) -> (-5.60165, 11.598282) centre (-4.922284, 13.45276) ccw
  arc A200 (-6.401854, 12.144517) -> (-6.74709, 12.20409) centre (-6.611616, 11.959045) ccw
  arc A201 (-6.74709, 12.20409) -> (-7.195507, 11.945196) centre (0, 0) ccw
  arc A202 (-7.195507, 11.945196) -> (-7.316534, 11.616427) centre (-7.051029, 11.70535) ccw
  arc A203 (-7.243582, 10.650312) -> (-7.316534, 11.616427) centre (-9.18929, 10.989203) ccw
  arc A204 (-7.305974, 10.552723) -> (-7.243582, 10.650312) centre (-7.391357, 10.676051) ccw
  arc A205 (-7.305974, 10.552723) -> (-7.778566, 10.209365) centre (0, 0) ccw
  arc A206 (-7.890659, 10.180183) -> (-7.778566, 10.209365) centre (-7.869473, 10.32868) ccw
  arc A207 (-8.786945, 10.54811) -> (-7.890659, 10.180183) centre (-7.611706, 12.135384) ccw
  arc A208 (-8.786945, 10.54811) -> (-9.137023, 10.534602) centre (-8.953562, 10.323079) ccw
  arc A209 (-9.137023, 10.534602) -> (-9.521813, 10.188135) centre (0, 0) ccw
  arc A210 (-9.521813, 10.188135) -> (-9.571841, 9.841387) centre (-9.330626, 9.983569) ccw
  arc A211 (-9.299617, 8.911552) -> (-9.571841, 9.841387) centre (-11.273265, 8.838502) ccw
  arc A212 (-9.340355, 8.803124) -> (-9.299617, 8.911552) centre (-9.449514, 8.906004) ccw
  arc A213 (-9.340355, 8.803124) -> (-9.731232, 8.369011) centre (0, 0) ccw
  arc A214 (-9.834808, 8.317162) -> (-9.731232, 8.369011) centre (-9.844959, 8.466818) ccw
  arc A215 (-10.788005, 8.4907) -> (-9.834808, 8.317162) centre (-9.968461, 10.287634) ccw
  arc A216 (-10.788005, 8.4907) -> (-11.127624, 8.404702) centre (-10.904194, 8.235945) ccw
  arc A217 (-11.127624, 8.404702) -> (-11.431971, 7.985803) centre (0, 0) ccw
  arc A218 (-11.431971, 7.985803) -> (-11.408813, 7.636232) centre (-11.20243, 7.825457) ccw
  arc A219 (-10.949214, 6.783314) -> (-11.408813, 7.636232) centre (-12.864545, 6.301516) ccw
  arc A220 (-10.966518, 6.668785) -> (-10.949214, 6.783314) centre (-11.094682, 6.746722) ccw
  arc A221 (-10.966518, 6.668785) -> (-11.258597, 6.162891) centre (0, 0) ccw
  arc A222 (-11.349129, 6.09064) -> (-11.258597, 6.162891) centre (-11.390174, 6.234915) ccw
  arc A223 (-12.317577, 6.062206) -> (-11.349129, 6.09064) centre (-11.889545, 7.990265) ccw
  arc A224 (-12.317577, 6.062206) -> (-12.631894, 5.907476) centre (-12.37826, 5.78886) ccw
  arc A225 (-12.631894, 5.907476) -> (-12.842497, 5.434454) centre (0, 0) ccw
  arc A226 (-12.842497, 5.434454) -> (-12.747164, 5.097336) centre (-12.584634, 5.325336) ccw
  arc A227 (-12.120277, 4.358613) -> (-12.747164, 5.097336) centre (-13.893583, 3.489123) ccw
  arc A228 (-12.113392, 4.242989) -> (-12.120277, 4.358613) centre (-12.254959, 4.292576) ccw
  arc A229 (-12.113392, 4.242989) -> (-12.293906, 3.687423) centre (0, 0) ccw
  arc A230 (-12.367439, 3.597928) -> (-12.293906, 3.687423) centre (-12.437583, 3.730517) ccw
  arc A231 (-13.308812, 3.368764) -> (-12.367439, 3.597928) centre (-13.291, 5.343683) ccw
  arc A232 (-13.308812, 3.368764) -> (-13.58409, 3.152065) centre (-13.311337, 3.088775) ccw
  arc A233 (-13.58409, 3.152065) -> (-13.691744, 2.645593) centre (0, 0) ccw
  arc A234 (-13.691744, 2.645593) -> (-13.528404, 2.335663) centre (-13.416829, 2.592472) ccw
  arc A235 (-12.761627, 1.74342) -> (-13.528404, 2.335663) centre (-14.315404, 0.524239) ccw
  arc A236 (-12.730852, 1.631754) -> (-12.761627, 1.74342) centre (-12.879635, 1.650824) ccw
  arc A237 (-12.730852, 1.631754) -> (-12.791913, 1.050797) centre (0, 0) ccw
  arc A238 (-12.845232, 0.94797) -> (-12.791913, 1.050797) centre (-12.94141, 1.063078) ccw
  arc A239 (-13.718388, 0.52809) -> (-12.845232, 0.94797) centre (-14.111574, 2.463557) ccw
  arc A240 (-13.718388, 0.52809) -> (-13.942597, 0.258894) centre (-13.662645, 0.253695) ccw
  constraints: 480 point on circle, 241 centre point
extrude "Extrusion1" cut sketch "_____6" along normal blind 11
sketch "_____10" plane through (0, 0, 0) normal (1, 0, 0) x (0, 0, -1)
  line L0 (-1.5, 6.4) -> (-1.5, 0)
  line L1 (-1.5, 0) -> (1.5, 0)
  line L2 (1.5, 0) -> (1.5, 6.4)
  line L3 (1.5, 6.4) -> (-1.5, 6.4)
  constraints: 8 end point
extrude "Extrusion2" cut sketch "_____10" along normal blind 15
sketch "_____18" plane through (7.5, 0, 0) normal (1, 0, 0) x (0, 0, -1)
  line L0 (0, 0) -> (0, 13.945)
  line L1 (0, 13.945) -> (1.621, 13.945)
  line L2 (1.621, 13.945) -> (1.621, 0)
  line L3 (1.621, 0) -> (0, 0)
  line L4 (0, 0) -> (0, 13.945)
  constraints: 10 end point
revolve "Revolution2" cut sketch "_____18" angle 360 about axis through (7.5, 0, 0) along (0, -1, 0)
thread "Thread1" size "M4x0.7" class "6H" standard "ISO Metric profile" length 8.945
sketch "_____19" plane through (7.5, 0, 0) normal (1, 0, 0) x (0, 0, -1)
  line L0 (0, 0) -> (12.076724, -6.9725)
  line L1 (12.076724, -6.9725) -> (11.266224, -8.376327)
  line L2 (11.266224, -8.376327) -> (-0.8105, -1.403827)
  line L3 (-0.8105, -1.403827) -> (0, 0)
  line L4 (0, 0) -> (12.076724, -6.9725)
  constraints: 10 end point
revolve "Revolution3" cut sketch "_____19" angle 360 about axis through (7.5, 0, 0) along (0, 0.5, 0.8660254)
thread "Thread2" size "M4x0.7" class "6H" standard "ISO Metric profile" length 8.945 offset 0.1755
ref_plane "to_belt_XY" through (7.5, 0, 0) normal (-1, 0, 0) x (0, 0, -1)
ref_plane "to_belt_YZ" through (7.5, 0, 0) normal (0, 0, -1) x (0, -1, 0)
ref_plane "to_belt_ZX" through (7.5, 0, 0) normal (0, -1, 0) x (-1, 0, 0)
ref_plane "to_screw1_XY" through (7.5, 6.4, 0) normal (0, 1, 0) x (1, 0, 0)
ref_plane "to_screw1_YZ" through (7.5, 6.4, 0) normal (1, 0, 0) x (0, 0, -1)
ref_plane "to_screw1_ZX" through (7.5, 6.4, 0) normal (0, 0, -1) x (0, 1, 0)
ref_plane "to_screw2_XY" through (7.5, -2.5, -4.330127) normal (0, -0.5, -0.8660254) x (1, 0, 0)
ref_plane "to_screw2_YZ" through (7.5, -2.5, -4.330127) normal (1, 0, 0) x (0, -0.8660254, 0.5)
ref_plane "to_screw2_ZX" through (7.5, -2.5, -4.330127) normal (0, -0.8660254, 0.5) x (0, -0.5, -0.8660254)
body "Solid1"
